Autodesk Fusion 360 part; units mm, degrees
(part 2 of 2)
  constraint tangent L309 A205
  constraint equal A152 A205
  constraint tangent L303 A206
  constraint tangent L302 A206
  constraint equal A152 A206
  constraint tangent L304 A207
  constraint tangent L303 A207
  constraint equal A152 A207
  constraint tangent L305 A208
  constraint tangent L304 A208
  constraint equal A152 A208
  constraint tangent L305 A209
  constraint tangent L306 A209
  constraint equal A152 A209
  constraint coincident P74 L306
  constraint coincident P74 L301
  constraint tangent L306 A210
  constraint tangent L301 A210
  constraint equal A152 A210
  constraint tangent L301 A211
  constraint tangent L302 A211
  constraint equal A152 A211
  constraint tangent L296 A212
  constraint tangent L297 A212
  constraint equal A152 A212
  constraint tangent L297 A213
  constraint tangent L298 A213
  constraint equal A152 A213
  constraint tangent L298 A214
  constraint tangent L299 A214
  constraint equal A152 A214
  constraint tangent L299 A215
  constraint tangent L300 A215
  constraint equal A152 A215
  constraint coincident P72 L300
  constraint coincident P72 L295
  constraint tangent L300 A216
  constraint tangent L295 A216
  constraint equal A152 A216
  constraint tangent L296 A217
  constraint tangent L295 A217
  constraint equal A152 A217
  constraint tangent L290 A218
  constraint tangent L291 A218
  constraint equal A152 A218
  constraint tangent L291 A219
  constraint tangent L292 A219
  constraint equal A152 A219
  constraint tangent L292 A220
  constraint tangent L293 A220
  constraint equal A152 A220
  constraint tangent L322 A221
  constraint tangent L321 A221
  constraint equal A152 A221
  constraint tangent L321 A222
  constraint tangent L320 A222
  constraint equal A152 A222
  constraint tangent L320 A223
  constraint tangent L319 A223
  constraint equal A152 A223
  constraint coincident P79 L319
  constraint coincident P79 L324
  constraint tangent L319 A224
  constraint tangent L324 A224
  constraint equal A152 A224
  constraint tangent L324 A225
  constraint tangent L323 A225
  constraint equal A152 A225
  constraint tangent L323 A226
  constraint tangent L322 A226
  constraint equal A152 A226
  constraint tangent L329 A227
  constraint tangent L328 A227
  constraint equal A152 A227
  constraint tangent L328 A228
  constraint tangent L327 A228
  constraint equal A152 A228
  constraint tangent L327 A229
  constraint tangent L326 A229
  constraint equal A152 A229
  constraint tangent L326 A230
  constraint tangent L325 A230
  constraint equal A152 A230
  constraint coincident P81 L325
  constraint coincident P81 L330
  constraint tangent L325 A231
  constraint tangent L330 A231
  constraint equal A152 A231
  constraint tangent L330 A232
  constraint tangent L329 A232
  constraint equal A152 A232
  constraint tangent L335 A233
  constraint tangent L334 A233
  constraint equal A152 A233
  constraint tangent L334 A234
  constraint tangent L333 A234
  constraint equal A152 A234
  constraint tangent L333 A235
  constraint tangent L332 A235
  constraint equal A152 A235
  constraint tangent L331 A236
  constraint tangent L332 A236
  constraint equal A152 A236
  constraint coincident P83 L331
  constraint coincident P83 L336
  constraint tangent L331 A237
  constraint tangent L336 A237
  constraint equal A152 A237
  constraint tangent L335 A238
  constraint tangent L336 A238
  constraint equal A152 A238
  constraint tangent L340 A239
  constraint tangent L341 A239
  constraint equal A152 A239
  constraint tangent L339 A240
  constraint tangent L340 A240
  constraint equal A152 A240
  constraint tangent L338 A241
  constraint tangent L339 A241
  constraint equal A152 A241
  constraint tangent L337 A242
  constraint tangent L338 A242
  constraint equal A152 A242
  constraint coincident P85 L337
  constraint coincident P85 L342
  constraint tangent L337 A243
  constraint tangent L342 A243
  constraint equal A152 A243
  constraint tangent L341 A244
  constraint tangent L342 A244
  constraint equal A152 A244
  constraint tangent L346 A245
  constraint tangent L347 A245
  constraint equal A152 A245
  constraint tangent L345 A246
  constraint tangent L346 A246
  constraint equal A152 A246
  constraint tangent L344 A247
  constraint tangent L345 A247
  constraint equal A152 A247
  constraint tangent L343 A248
  constraint tangent L344 A248
  constraint equal A152 A248
  constraint coincident P87 L343
  constraint coincident P87 L348
  constraint tangent L343 A249
  constraint tangent L348 A249
  constraint equal A152 A249
  constraint tangent L347 A250
  constraint tangent L348 A250
  constraint equal A152 A250
  constraint tangent L353 A251
  constraint tangent L354 A251
  constraint equal A152 A251
  constraint tangent L352 A252
  constraint tangent L353 A252
  constraint equal A152 A252
  constraint tangent L351 A253
  constraint tangent L352 A253
  constraint equal A152 A253
  constraint tangent L350 A254
  constraint tangent L351 A254
  constraint equal A152 A254
  constraint tangent L349 A255
  constraint tangent L350 A255
  constraint equal A152 A255
  constraint coincident P89 L349
  constraint coincident P89 L354
  constraint tangent L349 A256
  constraint tangent L354 A256
  constraint equal A152 A256
  constraint tangent L357 A257
  constraint tangent L358 A257
  constraint equal A152 A257
  constraint tangent L358 A258
  constraint tangent L359 A258
  constraint equal A152 A258
  constraint tangent L359 A259
  constraint tangent L360 A259
  constraint equal A152 A259
  constraint coincident P91 L355
  constraint coincident P91 L360
  constraint tangent L355 A260
  constraint tangent L360 A260
  constraint equal A152 A260
  constraint tangent L355 A261
  constraint tangent L356 A261
  constraint equal A152 A261
  constraint tangent L356 A262
  constraint tangent L357 A262
  constraint equal A152 A262
  constraint tangent L293 A263
  constraint tangent L294 A263
  constraint coincident P70 L289
  constraint coincident P70 L294
  constraint tangent L289 A264
  constraint tangent L294 A264
  constraint equal A263 A264
  constraint tangent L289 A265
  constraint tangent L290 A265
  constraint equal A263 A265
  measures "d1" diameter of A0
  measures "d3" distance of A0.centre L0.end
  measures "d6" radius of A1
  measures "d7" radius of A2
  measures "d8" radius of A4
  measures "d31" diameter of A121
  measures "d34" distance of A0.centre L240.end
  measures "d36" diameter of A122
  measures "d39" radius of A125
  measures "d52" diameter of A132
  measures "d55" diameter of A133
  measures "d56" diameter of A134
  measures "d59" diameter of A140
  measures "d62" diameter of A146
  measures "d68" distance of P58 P59
  measures "d69" distance of P60 P61
  measures "d70" distance of P62 P63
  measures "d71" distance of P64 P65
  measures "d72" distance of P66 P67
  measures "d73" distance of P68 P69
  measures "d74" distance of P70 P71
  measures "d75" distance of P72 P73
  measures "d76" distance of P74 A0.centre
  measures "d77" distance of P75 P76
  measures "d78" distance of P77 P78
  measures "d79" distance of P79 P80
  measures "d80" distance of P81 P82
  measures "d81" distance of P83 P84
  measures "d82" distance of P85 P86
  measures "d83" distance of P87 P88
  measures "d84" distance of P89 P90
  measures "d85" distance of P91 P92
  measures "d86" radius of A152
  measures "d87" radius of A263
extrude "Extrude3" add sketch "Stencil.Full.Hex" along normal blind 0.381 contours L241 L246 A129 A131 | L241 L242 A128 A131 | A131 | L245 L246 A130 A131 | L242 L243 A127 A131 | L244 L245 A125 A131 | L243 L244 A126 A131 makes body 1
extrude "Extrude4" add sketch "Stencil.Full.Hex" along normal blind 0.381 separate body contours L241 L246 A129 A131 | L241 L242 A128 A131 | L245 L246 A130 A131 | L242 L243 A127 A131 | L244 L245 A125 A131 | L243 L244 A126 A131 makes body 2 at (-23.3707, 0, 13.2774)
extrude "Extrude5" add sketch "Stencil.Full.Hex" along normal blind 0.762 contours A0 | A121 bodies 2
move_body "Move2" bodies 1 to x (1, 0, 0) y (0, 1, 0) z (0, 0, 1) at (0, 0.381, 0)
extrude "Extrude6" add sketch "Stencil.Full.Hex" along normal blind 1.762 contours A122 | A123 | A124 bodies 2
extrude "Extrude7" add 3 faces at (-30.5983, 1.762, 16.5684) (-0.8158, 1.762, -35.2169) (30.0235, 1.762, 16.5684) along direction (0, 1, 0) blind 0.6 on bodies 2 bodies 2
extrude "Extrude8" add sketch "Stencil.Full.Hex" along normal blind 2.362 contours A132 bodies 2
move_body "Move3" bodies 1 to x (1, 0, 0) y (0, 1, 0) z (0, 0, 1) at (0, 45, 0)
extrude "Extrude9" add sketch "Stencil.Full.Hex" along normal blind 0.381 separate body contours L6 L7 L8 L9 L10 L11 A1 A2 A3 A4 A5 A6 | L13 L14 L18 A7 L21 A8 L22 A9 A10 L23 A11 A12 | L25 L26 L30 A13 L33 A14 L34 A15 A16 L35 A17 A18 | L37 L38 L42 A19 L45 A20 L46 A21 A22 L47 A23 A24 | L49 L50 L54 A25 L57 A26 L58 A27 A28 L59 A29 A30 | L61 L62 L66 A31 L69 A32 L70 A33 A34 L71 A35 A36 A79 A80 L157 A81 A82 L160 L161 L164 L165 A83 L166 A84 | L73 L74 L78 A37 L81 A38 L82 A39 A40 L83 A41 A42 | L85 L86 L90 A43 L93 A44 L94 A45 A46 L95 A47 A48 | L97 L98 L102 A49 L105 A50 L106 A51 A52 L107 A53 A54 | L109 L110 L114 A55 L117 A56 L118 A57 A58 L119 A59 A60 | L121 L122 L126 A61 L129 A62 L130 A63 A64 L131 A65 A66 | A67 A68 L133 A69 A70 L136 L137 L140 L141 A71 L142 A72 | A73 A74 L145 A75 A76 L148 L149 L152 L153 A77 L154 A78 | A85 A86 L169 A87 A88 L172 L173 L176 L177 A89 L178 A90 | A91 A92 L181 A93 A94 L184 L185 L188 L189 A95 L190 A96 | L192 A97 A98 A99 A100 L198 L199 L200 L201 L203 A101 A102 | A103 A104 A105 L205 A106 L208 A107 L209 A108 L211 L212 L215 | A109 A110 L218 A111 L219 A112 L221 A113 L224 L225 A114 L227 | L228 L229 A115 L231 L232 A116 A117 L238 A118 A119 L239 A120 | L241 L246 A129 A131 | L241 L242 A128 A131 | A131 | L245 L246 A130 A131 | L242 L243 A127 A131 | L244 L245 A125 A131 | L243 L244 A126 A131 | L247 L248 L249 L250 L251 L252 A152 A153 A154 A155 A156 A157 | L253 L254 L255 L256 L257 L258 A158 A159 A160 A161 A162 A163 | L259 L260 L261 L262 L263 L264 A164 A165 A166 A167 A168 A169 | L265 L266 L267 L268 L269 L270 A170 A171 A172 A173 A174 A175 | L271 L272 L273 L274 L275 L276 A176 A177 A178 A179 A180 A181 | L277 L278 L279 L280 L281 L282 A182 A183 A184 A185 A186 A187 | L283 L284 L285 L286 L287 L288 A188 A189 A190 A191 A192 A193 | L289 L290 L291 L292 L293 L294 A218 A219 A220 A263 A264 A265 | L295 L296 L297 L298 L299 L300 A212 A213 A214 A215 A216 A217 | L301 L302 L303 L304 L305 L306 A206 A207 A208 A209 A210 A211 | L307 L308 L309 L310 L311 L312 A200 A201 A202 A203 A204 A205 | L313 L314 L315 L316 L317 L318 A194 A195 A196 A197 A198 A199 | L319 L320 L321 L322 L323 L324 A221 A222 A223 A224 A225 A226 | L325 L326 L327 L328 L329 L330 A227 A228 A229 A230 A231 A232 | L331 L332 L333 L334 L335 L336 A233 A234 A235 A236 A237 A238 | L337 L338 L339 L340 L341 L342 A239 A240 A241 A242 A243 A244 | L343 L344 L345 L346 L347 L348 A245 A246 A247 A248 A249 A250 | L349 L350 L351 L352 L353 L354 A251 A252 A253 A254 A255 A256 | L355 L356 L357 L358 L359 L360 A257 A258 A259 A260 A261 A262 makes body 3
move_body "Move4" bodies 3 to x (1, 0, 0) y (0, 1, 0) z (0, 0, 1) at (0, 0.381, 0)
move_body "Move5" bodies 3 to x (1, 0, 0) y (0, 1, 0) z (0, 0, 1) at (0, 22, 0)
extrude "Extrude10" add sketch "Stencil.Full.Hex" along normal blind 0.381 separate body contours L6 L7 L8 L9 L10 L11 A1 A2 A3 A4 A5 A6 | L13 L14 L18 A7 L21 A8 L22 A9 A10 L23 A11 A12 | L25 L26 L30 A13 L33 A14 L34 A15 A16 L35 A17 A18 | L37 L38 L42 A19 L45 A20 L46 A21 A22 L47 A23 A24 | L49 L50 L54 A25 L57 A26 L58 A27 A28 L59 A29 A30 | L61 L62 L66 A31 L69 A32 L70 A33 A34 L71 A35 A36 A79 A80 L157 A81 A82 L160 L161 L164 L165 A83 L166 A84 | L73 L74 L78 A37 L81 A38 L82 A39 A40 L83 A41 A42 | L85 L86 L90 A43 L93 A44 L94 A45 A46 L95 A47 A48 | L97 L98 L102 A49 L105 A50 L106 A51 A52 L107 A53 A54 | L109 L110 L114 A55 L117 A56 L118 A57 A58 L119 A59 A60 | L121 L122 L126 A61 L129 A62 L130 A63 A64 L131 A65 A66 | A67 A68 L133 A69 A70 L136 L137 L140 L141 A71 L142 A72 | A73 A74 L145 A75 A76 L148 L149 L152 L153 A77 L154 A78 | A85 A86 L169 A87 A88 L172 L173 L176 L177 A89 L178 A90 | A91 A92 L181 A93 A94 L184 L185 L188 L189 A95 L190 A96 | L192 A97 A98 A99 A100 L198 L199 L200 L201 L203 A101 A102 | A103 A104 A105 L205 A106 L208 A107 L209 A108 L211 L212 L215 | A109 A110 L218 A111 L219 A112 L221 A113 L224 L225 A114 L227 | L228 L229 A115 L231 L232 A116 A117 L238 A118 A119 L239 A120 | L241 L246 A129 A131 | L241 L242 A128 A131 | A131 | L245 L246 A130 A131 | L242 L243 A127 A131 | L244 L245 A125 A131 | L243 L244 A126 A131 makes body 4
move_body "Move6" bodies 4 to x (1, 0, 0) y (0, 1, 0) z (0, 0, 1) at (0, 0.381, 0)
move_body "Move7" bodies 4 to x (1, 0, 0) y (0, 1, 0) z (0, 0, 1) at (0, 33, 0)
move_body "Move8" bodies 3 to x (1, 0, 0) y (0, 1, 0) z (0, 0, 1) at (0, -15, 0)
move_body "Move9" bodies 4 to x (1, 0, 0) y (0, 1, 0) z (0, 0, 1) at (0, -11, 0)
move_body "Move10" bodies 1 to x (1, 0, 0) y (0, 1, 0) z (0, 0, 1) at (0, -8, 0)
move_body "Move11" bodies 3 4 1 to x (1, 0, 0) y (0, 1, 0) z (0, 0, 1) at (0, 8, 0)
copy_body "Body->Comp1" bodies 1 removing the originals makes body 5 in component "Stencil.Hex.Full"
copy_body "Body->Comp2" bodies 2 removing the originals makes body 6 in component "Holder"
copy_body "Body->Comp3" bodies 3 removing the originals makes body 7 in component "Stencil.Dot"
copy_body "Body->Comp4" bodies 4 removing the originals makes body 8 in component "Stencil.Hex.GND"
component "Stencil.Hex.Full" placed x (1, 0, 0) y (0, 1, 0) z (0, 0, 1) at (0, 0, 0)
component "Holder" placed x (1, 0, 0) y (0, 1, 0) z (0, 0, 1) at (0, 0, 0)
component "Stencil.Dot" placed x (1, 0, 0) y (0, 1, 0) z (0, 0, 1) at (0, 0, 0)
component "Stencil.Hex.GND" placed x (1, 0, 0) y (0, 1, 0) z (0, 0, 1) at (0, 0, 0)
named bodies: "Stencil.Hex.Full", "Holder", "Stencil.Dot", "Stencil.Hex.GND"
